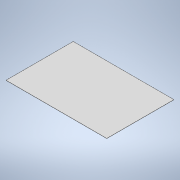
# Autodesk Inventor part: Suelo
Saved by Autodesk Inventor 2022 (Build 260153000, 153)
## iProperties
Created: 2023-04-08
Part Number: Suelo
Material: Genérico
Document SubType Name: Modeling
Designer: USUARIO
Density: 1 g/cm^3
Appearance: Valor por defecto
Author: USUARIO
Autodesk Inventor part; units mm, degrees
ref_plane "YZ Plane" through (0, 0, 0) normal (1, 0, 0) x (0, 1, 0)
ref_plane "XZ Plane" through (0, 0, 0) normal (0, 1, 0) x (-1, 0, 0)
ref_plane "XY Plane" through (0, 0, 0) normal (0, 0, 1) x (1, 0, 0)
sketch "Boceto1" plane through (0, 0, 0) normal (0, 1, 0) x (-1, 0, 0)
  line L0 (-3000, 2000) -> (3000, 2000)
  line L1 (3000, 2000) -> (3000, -2000)
  line L2 (3000, -2000) -> (-3000, -2000)
  line L3 (-3000, -2000) -> (-3000, 2000)
  line L4 (-3000, 2000) -> (3000, -2000) construction
  line L5 (3000, 2000) -> (-3000, -2000) construction
  point P0 (0, 0)
  dimension "d0" = 6000
  dimension "d1" = 4000
  constraints: 12 end point, 2 midpoint, 2 parallel, 1 horizontal, 1 perpendicular
  measures "d0" distance of L1.end L2.end
  measures "d1" distance of L0.end L1.end
extrude "Extrusión1" add sketch "Boceto1" along normal blind 10
